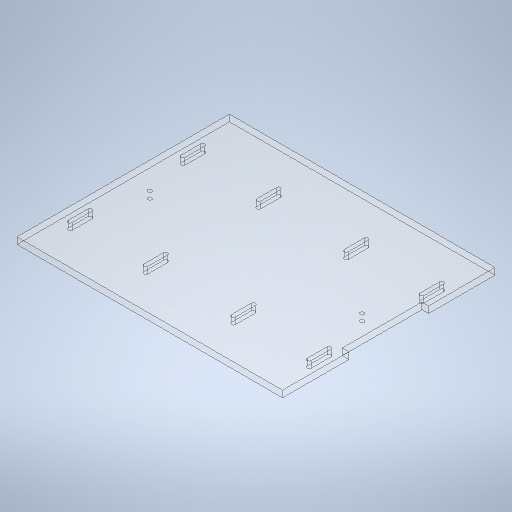
# Autodesk Inventor part: base_2
Saved by Autodesk Inventor 2025.3 (Build 293356030, 356C)
## iProperties
Created: 2026-06-26
Part Number: base_2
Material: Acrylic
Document SubType Name: Modeling
Designer: user
Density: 1.188 g/cm^3
Appearance: Transparent - Clear
Author: user
Autodesk Inventor part; units mm, degrees
ref_plane "YZ Plane" through (0, 0, 0) normal (1, 0, 0) x (0, 1, 0)
ref_plane "XZ Plane" through (0, 0, 0) normal (0, 1, 0) x (-1, 0, 0)
ref_plane "XY Plane" through (0, 0, 0) normal (0, 0, 1) x (1, 0, 0)
sketch "Sketch1" plane through (0, 0, 0) normal (0, 1, 0) x (-1, 0, 0)
  line L0 (0, 0) -> (-200, 0)
  line L1 (-200, 0) -> (-200, -160)
  line L2 (-200, -160) -> (0, -160)
  line L3 (85, -80) -> (-200, -80) construction
  line L4 (-100, 0) -> (-100, -160) construction
  line L5 (-38.5, 0) -> (-38.5, -160) construction
  line L6 (-123, 0) -> (-123, -160) construction
  line L7 (-10, -130) -> (-10, -115) construction
  line L8 (-10, -130) -> (-10, -115) construction
  line L9 (-8.5, -130) -> (-8.5, -115)
  line L10 (-11.5, -115) -> (-11.5, -130)
  arc A0 (-11.5, -130) -> (-8.5, -130) centre (-10, -130) ccw
  arc A1 (-8.5, -115) -> (-11.5, -115) centre (-10, -115) ccw
  line L11 (-67, -130) -> (-67, -115) construction
  line L12 (-67, -130) -> (-67, -115) construction
  line L13 (-68.5, -130) -> (-68.5, -115)
  line L14 (-65.5, -115) -> (-65.5, -130)
  arc A2 (-68.5, -130) -> (-65.5, -130) centre (-67, -130) ccw
  arc A3 (-65.5, -115) -> (-68.5, -115) centre (-67, -115) ccw
  line L15 (-120, -160) -> (-80, -160)
  line L16 (-80, -160) -> (-80, -155)
  line L17 (-80, -155) -> (-120, -155)
  line L18 (-120, -155) -> (-120, -160)
  line L19 (-190, -130) -> (-190, -115) construction
  line L20 (-190, -130) -> (-190, -115) construction
  line L21 (-191.5, -130) -> (-191.5, -115)
  line L22 (-188.5, -115) -> (-188.5, -130)
  arc A4 (-191.5, -130) -> (-188.5, -130) centre (-190, -130) ccw
  arc A5 (-188.5, -115) -> (-191.5, -115) centre (-190, -115) ccw
  line L23 (-134.5, -115) -> (-134.5, -130)
  line L24 (-133, -130) -> (-133, -115) construction
  line L25 (-131.5, -130) -> (-131.5, -115)
  arc A6 (-134.5, -130) -> (-131.5, -130) centre (-133, -130) ccw
  line L26 (-133, -130) -> (-133, -115) construction
  arc A7 (-131.5, -115) -> (-134.5, -115) centre (-133, -115) ccw
  line L27 (-100, -160) -> (-100, 0) construction
  line L28 (-10, -30) -> (-10, -45) construction
  line L29 (-10, -30) -> (-10, -45) construction
  line L30 (-8.5, -30) -> (-8.5, -45)
  line L31 (-11.5, -45) -> (-11.5, -30)
  arc A8 (-8.5, -30) -> (-11.5, -30) centre (-10, -30) ccw
  arc A9 (-11.5, -45) -> (-8.5, -45) centre (-10, -45) ccw
  line L32 (-65.5, -45) -> (-65.5, -30)
  line L33 (-67, -30) -> (-67, -45) construction
  line L34 (-68.5, -30) -> (-68.5, -45)
  arc A10 (-65.5, -30) -> (-68.5, -30) centre (-67, -30) ccw
  line L35 (-67, -30) -> (-67, -45) construction
  arc A11 (-68.5, -45) -> (-65.5, -45) centre (-67, -45) ccw
  line L36 (-120, 0) -> (-80, 0)
  line L37 (-80, 0) -> (-80, -5)
  line L38 (-80, -5) -> (-120, -5)
  line L39 (-120, -5) -> (-120, 0)
  arc A12 (-188.5, -30) -> (-191.5, -30) centre (-190, -30) ccw
  line L40 (-188.5, -45) -> (-188.5, -30)
  line L41 (-190, -30) -> (-190, -45) construction
  line L42 (-190, -30) -> (-190, -45) construction
  arc A13 (-191.5, -45) -> (-188.5, -45) centre (-190, -45) ccw
  line L43 (-191.5, -30) -> (-191.5, -45)
  line L44 (-134.5, -45) -> (-134.5, -30)
  line L45 (-133, -30) -> (-133, -45) construction
  line L46 (-133, -30) -> (-133, -45) construction
  arc A14 (-134.5, -45) -> (-131.5, -45) centre (-133, -45) ccw
  line L47 (-131.5, -30) -> (-131.5, -45)
  arc A15 (-131.5, -30) -> (-134.5, -30) centre (-133, -30) ccw
  line L48 (-200, -12.5) -> (-200, -62.5)
  line L49 (-200, -62.5) -> (-200, -110)
  line L50 (-200, -110) -> (-195, -110)
  line L51 (-195, -110) -> (-195, -50)
  line L52 (-195, -50) -> (-200, -50)
  line L53 (-200, -50) -> (-200, -12.5)
  line L54 (0, -160) -> (0, 0)
  point P0 (-10, -122.5)
  point P1 (-67, -122.5)
  point P2 (-190, -122.5)
  point P3 (-133, -122.5)
  point P4 (-10, -37.5)
  point P5 (-67, -37.5)
  point P6 (-190, -37.5)
  point P7 (-133, -37.5)
  point P8 (-67, -122.5)
  point P9 (-10, -122.5)
  point P10 (-120, -160)
  point P11 (-80, -160)
  point P12 (-80, 0)
  point P13 (-120, 0)
  point P14 (-190, -122.5)
  dimension "d2" = 15
  dimension "d4" = 30
  dimension "d6" = 1.5
  dimension "d9" = 40
  dimension "d13" = 0
  dimension "d14" = 5
  dimension "d16" = 20
  dimension "d22" = 5
  dimension "d26" = 30
  dimension "d27" = 30
  dimension "d28" = 0
  dimension "d30" = 160
  dimension "d32" = 57
  dimension "d56" = 10
  dimension "d57" = 200
  constraints: 126 end point, 55 symmetric about line, 32 point on circle, 16 centre point, 7 midpoint, 5 equal length, 5 perpendicular, 5 point on line, 4 tangent, 2 horizontal, 1 vertical, 14 other
  measures "d2" distance of L7.start L7.end
  measures "d4" distance from line of L2 L7.start
  measures "d6" radius of A0
  measures "d9" distance of L17.end L16.end
  measures "d13" distance between parallel lines of L2 L15
  measures "d14" distance between parallel lines of L17 L15
  measures "d16" distance between parallel lines of L4 L18
  measures "d22" distance between parallel lines of L49 L51
  measures "d26" distance between parallel lines of L3 L52
  measures "d27" distance between parallel lines of L3 L50
  measures "d28" distance between parallel lines of L1 L48
  measures "d30" distance between parallel lines of L0 L2
  measures "d32" distance of point (-67, -122.5) point (-10, -122.5)
  measures "d56" distance from line of L1 point (-190, -122.5)
  measures "d57" distance between parallel lines of L1 L54
extrude "Extrusion1" add sketch "Sketch1" along normal blind 5 contours L54 L2 L16 L17 L18 L1 L50 L51 L52 L0 L39 L38 L37 | L37 L38 L39 L0 | L2 L18 L17 L16
sketch "Sketch4" plane through (0, 5, 0) normal (0, 1, 0) x (1, 0, 0)
  line L0 (0, 0) -> (200, 0) projected
  line L1 (0, 160) -> (0, 0) projected
  point P0 (20, 80)
  dimension "d76" = 80
  dimension "d77" = 20
  measures "d76" distance from line of L0 point (20, 80)
  measures "d77" distance from line of L1 point (20, 80)
hole "Hole3" at (20, 5, -80) direction (0, -1, 0) diameter 3 end through all
sketch "Sketch5" plane through (0, 5, 0) normal (0, 1, 0) x (1, 0, 0)
  line L0 (195, 50) -> (195, 110) projected
  point P0 (0, 0)
  point P1 (180, 80)
  dimension "d85" = 15
  dimension "d86" = 30
  measures "d85" distance from line of L0 point (180, 80)
  measures "d86" vertical distance of point (180, 80) L0.end
hole "Hole4" at (180, 5, -80) direction (0, -1, 0) diameter 3 end through all
body "Solid1"
